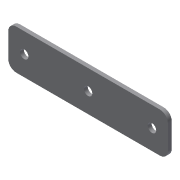
# Autodesk Inventor part: Super1
Saved by Autodesk Inventor 2015 SP1 (Build 190203100, 203)
## iProperties
Created: 2015-01-19
Part Number: Super1
Material: Generic
Document SubType Name: Sheet Metal
Designer: Owner
Density: 1 g/cm^3
Sheet Metal Rule: Default
Appearance: Default
Author: Owner
Autodesk Inventor part; units mm, degrees
ref_plane "YZ Plane" through (0, 0, 0) normal (1, 0, 0) x (0, 1, 0)
ref_plane "XZ Plane" through (0, 0, 0) normal (0, 1, 0) x (-1, 0, 0)
ref_plane "XY Plane" through (0, 0, 0) normal (0, 0, 1) x (1, 0, 0)
sketch "Sketch1" plane through (0, 0, 0) normal (0, 0, 1) x (1, 0, 0)
  line L0 (0, 0) -> (127, 0)
  line L1 (127, 0) -> (127, 31.75)
  line L2 (127, 31.75) -> (0, 31.75)
  line L3 (0, 31.75) -> (0, 0)
  circle A0 centre (114.3, 15.875) radius 3.3655
  circle A1 centre (63.5, 15.875) radius 3.3655
  circle A2 centre (12.7, 15.875) radius 3.3655
  dimension "d0" = 127
  dimension "d1" = 31.75
  dimension "d2" = 6.731
  dimension "d3" = 12.7
  dimension "d4" = 15.875
  dimension "d7" = 50.8
  measures "d0" distance of L2.end L1.end
  measures "d1" distance between parallel lines of L2 L0
  measures "d2" diameter of A0
  measures "d3" distance from line of A0.centre L1
  measures "d4" distance from line of A0.centre L2
  measures "d7" distance of A0.centre A1.centre
extrude "Plate1" add sketch "Sketch1" along normal blind 3.048
fillet "Corner Round1" radius 6.35 4 edges at (0, 31.75, 1.524) (0, 0, 1.524) (127, 31.75, 1.524) (127, 0, 1.524)
equation "\"d4\" = 0.5 * d1"
equation "\"BendRadius\" = Thickness"
equation "\"BendReliefWidth\" = Thickness"
equation "\"BendReliefDepth\" = 0.5 * Thickness"
equation "\"CornerReliefSize\" = 4 * Thickness"
equation "\"MinimumRemnant\" = 2 * Thickness"
equation "\"TransitionRadius\" = BendRadius"
equation "\"JacobiRadiusSize\" = BendRadius"
equation "\"GapSize\" = Thickness"
equation "\"d12\" = BendRadius"
equation "\"Thickness\" = 3.048"
body "Solid1"
